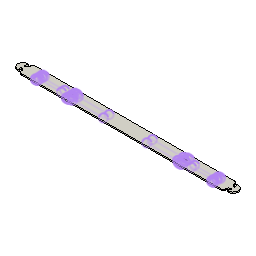
forehead_band (Autodesk Fusion 360 design; units mm, degrees)
Autodesk Fusion 360 part; units mm, degrees
sketch "Base" plane through (0, 0, 0) normal (0, 0, 1) x (1, 0, 0)
  arc A0 (-170, 8) -> (-170, -8) centre (-170, 0) ccw
  line L0 (-170, 8) -> (-170, 2.5)
  line L1 (-170, -8) -> (-170, -2.5)
  line L2 (-170, 2.5) -> (-169, 2.5)
  line L3 (-170, -2.5) -> (-169, -2.5)
  line L4 (-161, 11) -> (161, 11)
  line L5 (-161, -11) -> (161, -11)
  arc A1 (-169, 2.5) -> (-165, 6.75) centre (-169, 6.5074) ccw
  arc A2 (-161, 11) -> (-165, 6.75) centre (-161, 6.9926) ccw
  arc A3 (-165, -6.75) -> (-169, -2.5) centre (-169, -6.5074) ccw
  arc A4 (-165, -6.75) -> (-161, -11) centre (-161, -6.9926) ccw
  arc A5 (170, -8) -> (170, 8) centre (170, 0) ccw
  line L6 (170, 8) -> (170, 2.5) construction
  line L7 (170, 2.5) -> (169, 2.5)
  line L8 (170, -8) -> (170, -2.5) construction
  line L9 (170, -2.5) -> (169, -2.5)
  arc A6 (165, 6.75) -> (169, 2.5) centre (169, 6.5074) ccw
  arc A7 (165, 6.75) -> (161, 11) centre (161, 6.9926) ccw
  arc A8 (161, -11) -> (165, -6.75) centre (161, -6.9926) ccw
  arc A9 (169, -2.5) -> (165, -6.75) centre (169, -6.5074) ccw
  line L10 (-161, 11) -> (-161, -11) construction
  line L11 (-170, 2.5) -> (-170, -2.5) construction
  line L12 (-169, 2.5) -> (-169, -2.5) construction
  line L13 (-170, 8) -> (-170, -8) construction
  line L14 (-170, 0) -> (-169, 0) construction
  line L15 (-169, 0) -> (-161, 0) construction
  line L16 (-161, 0) -> (0, 0) construction
  line L17 (170, 8) -> (170, -8) construction
  line L18 (170, -2.5) -> (170, 2.5) construction
  line L19 (169, 2.5) -> (169, -2.5) construction
  line L20 (161, -11) -> (161, 11) construction
  line L21 (170, 0) -> (169, 0) construction
  line L22 (169, 0) -> (161, 0) construction
  line L23 (0, 0) -> (161, 0) construction
  line L24 (-168, 8) -> (-170, 8)
  line L25 (-168, -8) -> (-170, -8)
  arc A10 (-168, 8) -> (-170, 2.5) centre (-161.4375, 2.5) ccw
  arc A11 (-170, -2.5) -> (-168, -8) centre (-161.4375, -2.5) ccw
  line L26 (168, -8) -> (170, -8)
  line L27 (168, 8) -> (170, 8)
  arc A12 (170, 2.5) -> (168, 8) centre (161.4375, 2.5) ccw
  arc A13 (168, -8) -> (170, -2.5) centre (161.4375, -2.5) ccw
  point P0 (-161, 0)
  point P1 (-170, 0)
  point P2 (-169, 0)
  point P3 (161, 0)
  point P4 (169, 0)
  point P5 (170, 0)
  point P6 (170, 0)
  point P7 (-178, 0)
  dimension "d284" = 22
  dimension "d287" = 5
  dimension "d289" = 1
  dimension "d290" = 8
  dimension "d292" = 170
  dimension "d293" = 2
  dimension "d294" = 2
  dimension "d309" = 5.5
  constraint perpendicular L0 L2
  constraint perpendicular L1 L3
  constraint horizontal L5
  constraint horizontal L4
  constraint tangent L2 A1
  constraint tangent L4 A2
  constraint tangent A1 A2
  constraint equal A1 A2
  constraint tangent L3 A3
  constraint tangent L5 A4
  constraint tangent A3 A4
  constraint equal A3 A4
  constraint perpendicular L6 L7
  constraint perpendicular L8 L9
  constraint tangent L7 A6
  constraint tangent A6 A7
  constraint tangent L4 A7
  constraint equal A6 A7
  constraint tangent L9 A9
  constraint tangent L5 A8
  constraint coincident L5.end A8.start
  constraint tangent A8 A9
  constraint equal A8 A9
  constraint coincident A2 L4.start
  constraint coincident L4.start L10
  constraint midpoint L10 P0
  constraint midpoint L11 P1
  constraint vertical L10
  constraint vertical L11
  constraint perpendicular L3 L11
  constraint perpendicular L2 L11
  constraint perpendicular L3 L12
  constraint midpoint L12 P2
  constraint coincident P1 A0.centre
  constraint coincident P2 L14.end
  constraint coincident P0 L15.end
  constraint perpendicular L10 L15
  constraint coincident L16.end L23.start
  constraint parallel L5 L16
  constraint vertical L17
  constraint perpendicular L7 L18
  constraint perpendicular L9 L19
  constraint perpendicular L4 L20
  constraint midpoint L20 P3
  constraint midpoint L19 P4
  constraint midpoint L18 P6
  constraint coincident P6 P5
  constraint midpoint P6 L17
  constraint coincident P4 L21.end
  constraint perpendicular L19 L21
  constraint coincident P3 L22.end
  constraint perpendicular L20 L22
  constraint equal L16 L23
  constraint equal L15 L22
  constraint equal L14 L21
  constraint equal L13 L17
  constraint equal L11 L18
  constraint tangent L0 A10
  constraint tangent L1 A11
  constraint tangent L6 A12
  constraint tangent L8 A13
  constraint coincident L24.start A10.start
  constraint coincident L25.start A11.end
  constraint equal L24 L27
  constraint equal L26 L27
  constraint coincident L26.start A13.start
  constraint coincident L27.start A12.end
  constraint midpoint A0 P7
  constraint coincident A0.centre L14.start
  constraint coincident A0.end L1.start
  constraint horizontal L24
  constraint horizontal L25
  constraint coincident A5.end L6.start
  constraint coincident A5.start L8.start
  constraint horizontal L27
  constraint horizontal L26
  constraint equal L0 L1
  constraint coincident A0.start L0.start
  constraint coincident L24.start L27
  measures "d284" distance of L4.start L5.start
  measures "d287" distance of L0.end L1.end
  measures "d289" distance of P1 P2
  measures "d290" distance of P2 P0
  measures "d292" horizontal distance of L16.end A0.end
  measures "d293" distance of A0.start L24.start
  measures "d294" distance of A0.end L25.start
  measures "d309" distance of A0.start L0.end
extrude "Extrude3" add sketch "Base" along normal blind 2
sketch "Shield Connector" plane through (0, 0, 0) normal (0, 0, 1) x (1, 0, 0)
  line L0 (-105, 2.5) -> (-141, 2.5)
  line L1 (-141, 2.5) -> (-141, 5.5)
  line L2 (-141, 5.5) -> (-144, 5.5)
  line L3 (-144, -5.5) -> (-141, -5.5)
  line L4 (-141, -5.5) -> (-141, -2.5)
  line L5 (-141, -2.5) -> (-105, -2.5)
  arc A0 (-144, 5.5) -> (-144, -5.5) centre (-144, 0) ccw
  line L6 (105, 2.5) -> (141, 2.5)
  line L7 (141, 2.5) -> (141, 5.5)
  line L8 (141, 5.5) -> (144, 5.5)
  line L9 (144, -5.5) -> (141, -5.5)
  line L10 (141, -5.5) -> (141, -2.5)
  line L11 (141, -2.5) -> (105, -2.5)
  arc A1 (144, -5.5) -> (144, 5.5) centre (144, 0) ccw
  line L12 (-141, 2.5) -> (-141, -2.5) construction
  line L13 (-105, 2.5) -> (-105, -2.5) construction
  line L14 (-144, 5.5) -> (-144, -5.5) construction
  line L15 (-144, 0) -> (0, 0) construction
  line L16 (0, 0) -> (144, 0) construction
  point P0 (-141, 0)
  point P1 (-105, 0)
  dimension "d270" = 105
  dimension "d271" = 36
  dimension "d272" = 3
  dimension "d273" = 5
  dimension "d274" = 11
  constraint horizontal L0
  constraint perpendicular L0 L1
  constraint perpendicular L1 L2
  constraint horizontal L3
  constraint perpendicular L3 L4
  constraint perpendicular L4 L5
  constraint perpendicular L6 L7
  constraint perpendicular L7 L8
  constraint parallel L8 L9
  constraint perpendicular L8 L10
  constraint perpendicular L10 L11
  constraint coincident L9.start A1.start
  constraint coincident A0.centre L15.start
  constraint coincident L15.end L16.start
  constraint perpendicular L13 L15
  constraint midpoint L12 P0
  constraint midpoint L13 P1
  constraint coincident L15 P0
  constraint coincident L15 P1
  constraint midpoint A0.centre L14
  constraint coincident L3 A0.end
  constraint coincident L0.start L6
  constraint coincident L5.end L11
  constraint coincident L3.end L9
  constraint coincident L1.end L8
  constraint equal L5 L11
  constraint coincident A1.centre L16.end
  constraint perpendicular L10 L16
  constraint equal L15 L16
  constraint equal L3 L9
  constraint equal L6 L11
  constraint equal L8 L9
  constraint vertical L7
  measures "d270" distance of L15.end L13
  measures "d271" distance of L12 L13
  measures "d272" distance of L3.end L3.start
  measures "d273" distance of L0.start L5.end
  measures "d274" distance of L2.end L3.start
sketch "Frame Connector" plane through (0, 0, 0) normal (0, 0, 1) x (1, 0, 0)
  line L0 (-35, 0) -> (35, 0) construction
  line L1 (-85, 0) -> (85, 0) construction
  line L2 (-85, 4.5) -> (-35, 4.5)
  line L3 (-85, -4.5) -> (-35, -4.5)
  line L4 (-35, 4.5) -> (-35, -4.5) construction
  line L5 (-85, 4.5) -> (-85, -4.5) construction
  line L6 (35, 4.5) -> (85, 4.5)
  line L7 (85, -4.5) -> (35, -4.5)
  line L8 (35, 4.5) -> (35, -4.5) construction
  line L9 (85, 4.5) -> (85, -4.5) construction
  line L10 (-85, 0) -> (-89, 0) construction
  line L11 (85, 0) -> (89, 0) construction
  line L12 (-94, 1.5) -> (-89, 1.5)
  line L13 (-89, 1.5) -> (-89, -1.5)
  line L14 (-89, -1.5) -> (-94, -1.5)
  line L15 (-94, -1.5) -> (-94, 1.5)
  line L16 (89, 1.5) -> (94, 1.5)
  line L17 (94, 1.5) -> (94, -1.5)
  line L18 (94, -1.5) -> (89, -1.5)
  line L19 (89, -1.5) -> (89, 1.5)
  line L20 (-89, 6.5) -> (-92.5, 6.5)
  line L21 (-89, -6.5) -> (-92.5, -6.5)
  line L22 (-89, 6.5) -> (-89, -6.5) construction
  line L23 (-92.5, 6.5) -> (-92.5, -6.5) construction
  arc A0 (-92.5, 6.5) -> (-92.5, -6.5) centre (-92.5, 0) ccw
  line L24 (89, 6.5) -> (89, -6.5) construction
  line L25 (89, 6.5) -> (92.5, 6.5)
  line L26 (89, -6.5) -> (92.5, -6.5)
  line L27 (92.5, 6.5) -> (92.5, -6.5) construction
  arc A1 (92.5, -6.5) -> (92.5, 6.5) centre (92.5, 0) ccw
  arc A2 (89, 6.5) -> (85, 4.5) centre (89, 1.5) ccw
  arc A3 (85, -4.5) -> (89, -6.5) centre (89, -1.5) ccw
  arc A4 (-85, 4.5) -> (-89, 6.5) centre (-89, 1.5) ccw
  arc A5 (-89, -6.5) -> (-85, -4.5) centre (-89, -1.5) ccw
  line L28 (-91.5, 1.5) -> (-91.5, -1.5) construction
  line L29 (-89, 0) -> (-91.5, 0)
  line L30 (91.5, 1.5) -> (91.5, -1.5) construction
  line L31 (89, 0) -> (91.5, 0)
  point P0 (-92.5, 0)
  point P1 (92.5, 0)
  dimension "d300" = 35
  dimension "d301" = 50
  dimension "d302" = 9
  dimension "d303" = 4
  dimension "d305" = 3
  dimension "d306" = 5
  dimension "d307" = 3.5
  dimension "d308" = 13
  constraint horizontal L0
  constraint midpoint origin L0
  constraint parallel L0 L1
  constraint midpoint origin L1
  constraint parallel L1 L2
  constraint parallel L1 L3
  constraint perpendicular L1 L4
  constraint perpendicular L3 L5
  constraint midpoint L0.start L4
  constraint midpoint L1.start L5
  constraint parallel L1 L6
  constraint parallel L1 L7
  constraint perpendicular L7 L8
  constraint coincident L0.end L8
  constraint coincident L1.end L9
  constraint perpendicular L7 L9
  constraint coincident L2.end L6
  constraint coincident L3.end L7
  constraint perpendicular L5 L10
  constraint perpendicular L9 L11
  constraint equal L10 L11
  constraint horizontal L12
  constraint vertical L13
  constraint horizontal L14
  constraint vertical L15
  constraint midpoint L10.end L13
  constraint horizontal L16
  constraint vertical L17
  constraint horizontal L18
  constraint vertical L19
  constraint midpoint L11.end L19
  constraint coincident L12.end L16
  constraint equal L14 L18
  constraint perpendicular L15 L20
  constraint horizontal L21
  constraint midpoint L10.end L22
  constraint parallel L13 L22
  constraint equal L20 L21
  constraint midpoint L23 P0
  constraint coincident P0 A0.centre
  constraint perpendicular L16 L24
  constraint midpoint L11.end L24
  constraint equal L22 L24
  constraint perpendicular L24 L25
  constraint perpendicular L24 L26
  constraint equal L20 L25
  constraint equal L25 L26
  constraint midpoint L27 P1
  constraint coincident P1 A1.centre
  constraint tangent L25 A2
  constraint tangent L26 A3
  constraint tangent L21 A5
  constraint tangent L20 A4
  constraint midpoint L12 L28.start
  constraint midpoint L14 L28.end
  constraint midpoint L28 L29.end
  constraint midpoint L16 L30.start
  constraint midpoint L18 L30.end
  constraint midpoint L30 L31.end
  measures "d300" distance of origin L0.start
  measures "d301" distance of L0.start L1.start
  measures "d302" distance of L2.start L3.start
  measures "d303" distance of L1.start L10.end
  measures "d305" distance of L12.end L13.end
  measures "d306" distance of L12.start L12.end
  measures "d307" distance of L21.start L21.end
  measures "d308" distance of L20.start L21.start
extrude "Extrude5" cut sketch "Frame Connector" along normal blind 2
sketch "Cuts" plane through (0, 0, 0) normal (0, 0, 1) x (1, 0, 0)
  line L0 (-141, -5.5) -> (-141, -2.5)
  line L1 (-144, -5.5) -> (-141, -5.5)
  line L2 (-141, -2.5) -> (-105, -2.5)
  line L3 (-141, 2.5) -> (-141, 5.5)
  line L4 (-141, 5.5) -> (-144, 5.5)
  arc A0 (-144, 5.5) -> (-144, -5.5) centre (-144, 0) ccw
  line L5 (-105, 2.5) -> (-141, 2.5)
  line L6 (144, -5.5) -> (141, -5.5)
  line L7 (141, -5.5) -> (141, -2.5)
  line L8 (141, -2.5) -> (105, -2.5)
  line L9 (141, 2.5) -> (141, 5.5)
  line L10 (141, 5.5) -> (144, 5.5)
  arc A1 (144, -5.5) -> (144, 5.5) centre (144, 0) ccw
  line L11 (105, 2.5) -> (141, 2.5)
  line L12 (-85, -4.5) -> (-35, -4.5)
  arc A2 (-89, -6.5) -> (-85, -4.5) centre (-89, -1.5) ccw
  line L13 (-89, -6.5) -> (-92.5, -6.5)
  arc A3 (-92.5, 6.5) -> (-92.5, -6.5) centre (-92.5, 0) ccw
  line L14 (-89, 6.5) -> (-92.5, 6.5)
  arc A4 (-85, 4.5) -> (-89, 6.5) centre (-89, 1.5) ccw
  line L15 (-85, 4.5) -> (-35, 4.5)
  arc A5 (89, 6.5) -> (85, 4.5) centre (89, 1.5) ccw
  line L16 (89, 6.5) -> (92.5, 6.5)
  arc A6 (92.5, -6.5) -> (92.5, 6.5) centre (92.5, 0) ccw
  line L17 (89, -6.5) -> (92.5, -6.5)
  arc A7 (85, -4.5) -> (89, -6.5) centre (89, -1.5) ccw
  line L18 (85, -4.5) -> (35, -4.5)
  line L19 (35, 4.5) -> (85, 4.5)
  line L20 (-89, 0) -> (-91.5, 0)
  line L21 (89, 0) -> (91.5, 0)
named bodies: "Main body"
